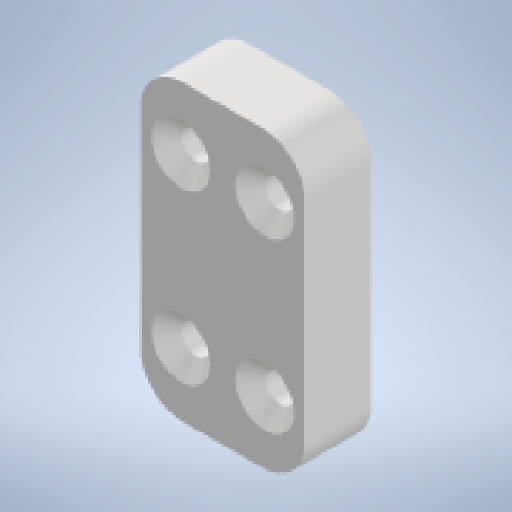
# Autodesk Inventor part: RailTab
Saved by Autodesk Inventor 2023.1 (Build 271208000, 208)
## iProperties
Created: 2023-06-05
Part Number: RailTab
Material: Generic
Document SubType Name: Modeling
Designer: hello
Density: 1 g/cm^3
Appearance: Default
Author: hello
Autodesk Inventor part; units mm, degrees
ref_plane "YZ Plane" through (0, 0, 0) normal (1, 0, 0) x (0, 1, 0)
ref_plane "XZ Plane" through (0, 0, 0) normal (0, 1, 0) x (-1, 0, 0)
ref_plane "XY Plane" through (0, 0, 0) normal (0, 0, 1) x (1, 0, 0)
sketch "Sketch1" plane through (0, 0, 0) normal (0, 0, 1) x (1, 0, 0)
  line L0 (-9.75, 17.5) -> (9.75, 17.5)
  line L1 (9.75, 17.5) -> (9.75, -17.5)
  line L2 (9.75, -17.5) -> (-9.75, -17.5)
  line L3 (-9.75, -17.5) -> (-9.75, 17.5)
  line L4 (-9.75, 17.5) -> (9.75, -17.5) construction
  line L5 (9.75, 17.5) -> (-9.75, -17.5) construction
  point P0 (0, 0)
  dimension "d0" = 19.5
  dimension "d1" = 35
  constraints: 12 end point, 2 midpoint, 2 parallel, 1 horizontal, 1 perpendicular
  measures "d0" distance of L1.end L2.end
  measures "d1" distance of L0.end L1.end
extrude "Extrusion1" add sketch "Sketch1" along normal blind 7.9
sketch "Sketch2" plane through (0, 0, 7.9) normal (0, 0, 1) x (1, 0, 0)
  line L0 (-5, 10) -> (5, 10)
  line L1 (5, 10) -> (5, -10)
  line L2 (5, -10) -> (-5, -10)
  line L3 (-5, -10) -> (-5, 10)
  line L4 (-5, 10) -> (5, -10) construction
  line L5 (5, 10) -> (-5, -10) construction
  point P0 (0, 0)
  dimension "d4" = 10
  dimension "d5" = 20
  constraints: 12 end point, 4 coincident, 2 midpoint, 2 parallel, 1 horizontal, 1 perpendicular
  measures "d4" distance of L1.end L2.end
  measures "d5" distance of L0.end L1.end
hole "Hole1" at (-5, 10, 7.9) at (5, 10, 7.9) at (5, -10, 7.9) at (-5, -10, 7.9) direction (0, 0, -1) diameter 3.4 end through all countersink diameter 8 countersink angle 90 clearance for "Countersunk Flat Head Screw ISO 2009/7046" size "M3" standard "ISO"
fillet "Fillet1" radius 5 4 edges at (9.75, -17.5, 3.95) (-9.75, -17.5, 3.95) (-9.75, 17.5, 3.95) (9.75, 17.5, 3.95)
body "Solid1"
